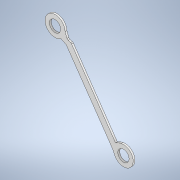
# Autodesk Inventor part: Pieza9
Saved by Autodesk Inventor 2022 (Build 260153000, 153)
## iProperties
Created: 2022-11-04
Part Number: Pieza9
Material: Resina acetálica, blanca
Document SubType Name: Modeling
Designer: Mauricio Guerrero
Density: 1.425 g/cm^3
Appearance: Suave - Blanco
Author: Mauricio Guerrero
Autodesk Inventor part; units mm, degrees
ref_plane "YZ Plane" through (0, 0, 0) normal (1, 0, 0) x (0, 1, 0)
ref_plane "XZ Plane" through (0, 0, 0) normal (0, 1, 0) x (-1, 0, 0)
ref_plane "XY Plane" through (0, 0, 0) normal (0, 0, 1) x (1, 0, 0)
sketch "Boceto1" plane through (0, 0, 0) normal (0, 0, 1) x (1, 0, 0)
  circle A0 centre (689.7833, 250.3365) radius 1.25
  arc A1 (692.0258, 250.3365) -> (691.1197, 248.5357) centre (689.7833, 250.3365) ccw
  circle A2 centre (705.0833, 232.8865) radius 1.25
  arc A3 (703.026, 232.2284) -> (704.5342, 234.9755) centre (705.0833, 232.8865) ccw
  line L0 (692.0258, 250.3365) -> (692.4482, 249.264)
  line L1 (692.7, 249.0291) -> (693.2607, 248.8522)
  line L2 (693.4693, 248.6983) -> (703.3196, 234.461)
  line L3 (704.0922, 234.8593) -> (704.5342, 234.9755)
  line L4 (691.1197, 248.5357) -> (692.1871, 248.0115)
  line L5 (692.3398, 247.8801) -> (702.6433, 232.9876)
  line L6 (702.665, 232.951) -> (703.026, 232.2284)
  arc A4 (702.665, 232.951) -> (702.6433, 232.9876) centre (702.3966, 232.8169) ccw
  arc A5 (692.4482, 249.264) -> (692.7, 249.0291) centre (692.8204, 249.4105) ccw
  arc A6 (692.3398, 247.8801) -> (692.1871, 248.0115) centre (692.0108, 247.6525) ccw
  arc A7 (693.4693, 248.6983) -> (693.2607, 248.8522) centre (693.1404, 248.4707) ccw
  line L7 (703.3196, 234.461) -> (703.3337, 234.4726)
  arc A8 (704.0922, 234.8593) -> (703.3337, 234.4726) centre (704.6006, 232.925) ccw
  point P0 (0, 0)
  dimension "d7" = 2.5
  dimension "d8" = 4.485
  dimension "d9" = 2.5
  dimension "d10" = 4.32
  dimension "d11" = 15.3
  dimension "d12" = 17.45
  dimension "d14" = 0.4
  dimension "d17" = 2
  constraints: 16 end point, 14 point on circle, 11 tangent, 9 centre point, 2 coincident, 2 equal radius, 1 parallel
  measures "d7" diameter of A0
  measures "d8" diameter of A1
  measures "d9" diameter of A2
  measures "d10" diameter of A3
  measures "d11" horizontal distance of A2.centre A0.centre
  measures "d12" vertical distance of A2.centre A0.centre
  measures "d14" radius of A5
  measures "d17" radius of A8
extrude "Extrusión1" add sketch "Boceto1" along normal blind 0.4
